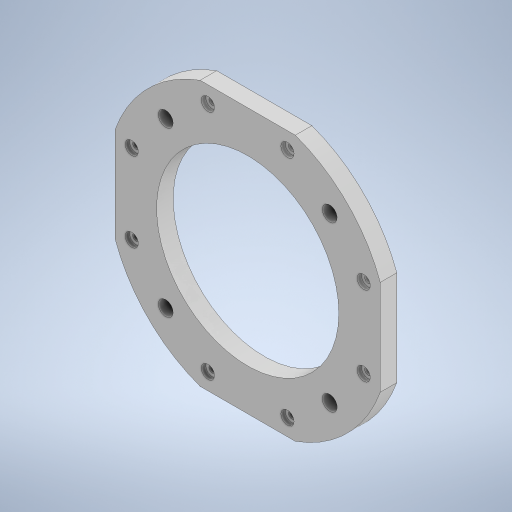
# Autodesk Inventor part: 감속기어1 - 하우징 커버
Saved by Autodesk Inventor 2023 (Build 270158000, 158)
## iProperties
Created: 2022-06-21
Part Number: 감속기어1 - 하우징 커버
Material: 일반
Document SubType Name: Modeling
Designer: user
Density: 1 g/cm^3
Appearance: 기본값
Author: user
Autodesk Inventor part; units mm, degrees
ref_plane "YZ Plane" through (0, 0, 0) normal (1, 0, 0) x (0, 1, 0)
ref_plane "XZ Plane" through (0, 0, 0) normal (0, 1, 0) x (-1, 0, 0)
ref_plane "XY Plane" through (0, 0, 0) normal (0, 0, 1) x (1, 0, 0)
sketch "스케치1" plane through (0, 0, 0) normal (0, 0, 1) x (1, 0, 0)
  circle A0 centre (0, 0) radius 42.5
  line L0 (-40, -40) -> (40, -40)
  line L1 (40, -40) -> (40, 40)
  line L2 (40, 40) -> (-40, 40)
  line L3 (-40, 40) -> (-40, -40)
  line L4 (-40, -40) -> (40, 40) construction
  line L5 (40, -40) -> (-40, 40) construction
  circle A1 centre (0, 0) radius 27.5
  point P0 (-40, 14.3614)
  point P1 (-40, -14.3614)
  point P2 (-14.3614, -40)
  point P3 (14.3614, -40)
  point P4 (40, -14.3614)
  point P5 (40, 14.3614)
  point P6 (14.3614, 40)
  point P7 (-14.3614, 40)
  dimension "d0" = 85
  dimension "d1" = 80
  dimension "d2" = 80
  dimension "d3" = 55
  constraints: 12 end point, 2 centre point, 2 coincident, 2 midpoint, 2 parallel, 1 horizontal, 1 perpendicular
  measures "d0" diameter of A0
  measures "d1" distance of L2.end L1.end
  measures "d2" distance of L1.end L0.end
  measures "d3" diameter of A1
extrude "돌출1" add sketch "스케치1" along normal blind 5 contours L1 A0 L0 L3 L2
sketch "스케치2" plane through (0, 0, 5) normal (0, 0, 1) x (1, 0, 0)
  circle A0 centre (-12, 35) radius 1
  line L0 (0, 0) -> (0, 47.7452)
  circle A1 centre (-12, 35) radius 2
  circle A2 centre (12, 35) radius 1
  circle A3 centre (12, 35) radius 2
  dimension "d6" = 2
  dimension "d7" = 35
  dimension "d8" = 12
  dimension "d9" = 4
  constraints: 4 centre point, 2 coincident, 2 end point, 2 symmetric about line, 1 vertical, 2 other
  measures "d6" diameter of A0
  measures "d7" vertical distance of L0.start A0.centre
  measures "d8" distance from line of L0 A0.centre
  measures "d9" diameter of A1
extrude "돌출2" cut sketch "스케치2" against normal blind 1.3 contours A0 | A1 | A2 | A3
extrude "돌출3" cut sketch "스케치2" against normal blind 10.5 contours A0 | A2
pattern_circular "원형 패턴1" count 4 over 360 about axis through (0, 0, 0) along (0, 0, 1) of "돌출2", "돌출3"
sketch "스케치3" plane through (0, 0, 5) normal (0, 0, 1) x (1, 0, 0)
  circle A0 centre (0, 0) radius 35 construction
  line L0 (0, 0) -> (-24.7487, 24.7487) construction
  line L1 (0, 0) -> (0, 35) construction
  circle A1 centre (-24.7487, 24.7487) radius 2.25
  dimension "d17" = 70
  dimension "d18" = 45
  dimension "d19" = 4.5
  constraints: 4 end point, 2 centre point, 2 point on circle, 1 coincident, 1 vertical
  measures "d17" diameter of A0
  measures "d18" angle of L1 L0
  measures "d19" diameter of A1
extrude "돌출4" cut sketch "스케치3" against normal blind 5
pattern_circular "원형 패턴2" count 4 over 360 about axis through (0, 0, 0) along (0, 0, 1) of "돌출4"
